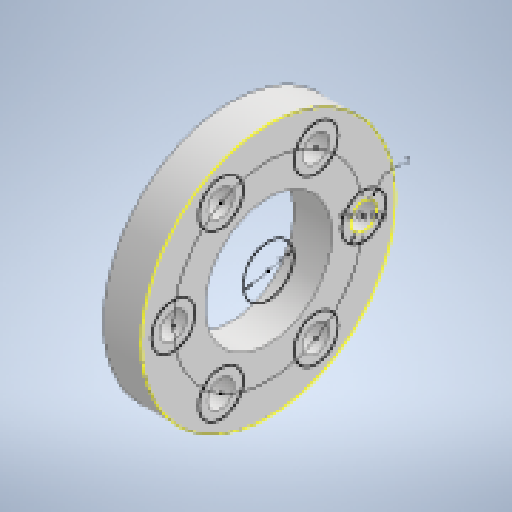
# Autodesk Inventor part: 链轮摇臂座
Saved by Autodesk Inventor 2025.1 (Build 291241000, 241)
## iProperties
Created: 2025-08-27
Part Number: 链轮摇臂座
Material: 常规
Document SubType Name: Modeling
Designer: Piw
Density: 1 g/cm^3
Appearance: 默认
Author: Piw
Autodesk Inventor part; units mm, degrees
ref_plane "YZ Plane" through (0, 0, 0) normal (1, 0, 0) x (0, 1, 0)
ref_plane "XZ Plane" through (0, 0, 0) normal (0, 1, 0) x (-1, 0, 0)
ref_plane "XY Plane" through (0, 0, 0) normal (0, 0, 1) x (1, 0, 0)
sketch "草图1" plane through (0, 0, 0) normal (1, 0, 0) x (0, 1, 0)
  circle A0 centre (0, 0) radius 15 construction
  line L0 (0, 0) -> (0, -15) construction
  circle A1 centre (0, 0) radius 10
  circle A2 centre (0, -15) radius 2.1
  circle A3 centre (12.9904, -7.5) radius 2.1
  circle A4 centre (12.9904, 7.5) radius 2.1
  circle A5 centre (0, 15) radius 2.1
  circle A6 centre (-12.9904, 7.5) radius 2.1
  circle A7 centre (-12.9904, -7.5) radius 2.1
  circle A8 centre (0, 0) radius 20
  dimension "d0" = 30
  dimension "d1" = 20
  dimension "d2" = 4.2
  dimension "d5" = 360
  dimension "d7" = 40
  constraints: 8 centre point, 4 coincident, 2 end point, 1 vertical, 1 vertical alignment, 15 other
  measures "d1" diameter of A1
  measures "d2" diameter of A2
  measures "d7" diameter of A8
extrude "拉伸1" add sketch "草图1" along normal blind 6
sketch "草图2" plane through (6, 0, 0) normal (1, 0, 0) x (0, 0, -1)
  circle A0 centre (0, 0) radius 4
  circle A1 centre (0, 0) radius 20 projected
  circle A2 centre (15, 0) radius 2.1 projected
  circle A3 centre (15, 0) radius 3.5
  circle A4 centre (7.5, 12.9904) radius 3.5
  circle A5 centre (-7.5, 12.9904) radius 3.5
  circle A6 centre (-15, 0) radius 3.5
  circle A7 centre (-7.5, -12.9904) radius 3.5
  circle A8 centre (7.5, -12.9904) radius 3.5
  dimension "d10" = 8
  dimension "d11" = 7
  dimension "d14" = 360
  constraints: 7 centre point, 2 coincident, 13 other
  measures "d10" diameter of A0
  measures "d11" diameter of A3
extrude "拉伸2" add sketch "草图2" along normal blind 5 contours A1
sketch "草图3" plane through (11, 0, 0) normal (1, 0, 0) x (0, 0, -1)
  circle A0 centre (0, 0) radius 4 projected
  circle A1 centre (0, 0) radius 9
  dimension "d18" = 18
  constraints: 1 centre point, 1 coincident
  measures "d18" diameter of A1
extrude "拉伸3" add sketch "草图3" along normal blind 10
chamfer "倒角1" distance 2 angle 45 1 edges at (11, 0, 9)
chamfer "倒角2" distance 1 angle 45 1 edges at (11, 0, 20)
